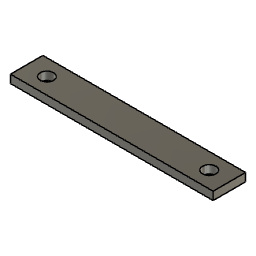
Headbar (Autodesk Fusion 360 design; units mm, degrees)
Autodesk Fusion 360 part; units mm, degrees
sketch "Sketch1" plane through (0, 0, 0) normal (0, 0, 1) x (1, 0, 0)
  line L0 (-47.1003, 10.1518) -> (-22.1003, 10.1518)
  line L1 (-22.1003, 10.1518) -> (-22.1003, 6.1518)
  line L2 (-22.1003, 6.1518) -> (-47.1003, 6.1518)
  line L3 (-47.1003, 6.1518) -> (-47.1003, 10.1518)
  circle A0 centre (-44.6003, 8.1518) radius 0.825
  circle A1 centre (-24.6003, 8.1696) radius 0.825
  line L4 (-47.1003, 8.1518) -> (-44.6003, 8.1518) construction
  line L5 (-22.1003, 8.1518) -> (-24.6003, 8.1696)
  dimension "d1" = 25
  dimension "d2" = 4
  dimension "d3" = 1.65
  dimension "d4" = 1.65
  dimension "d7" = 2.5
  dimension "d8" = 2.5
  constraint horizontal L0
  constraint vertical L1
  constraint horizontal L2
  constraint vertical L3
  constraint midpoint L3 L4.start
  constraint perpendicular L3 L4
  constraint coincident A0.centre L4.end
  constraint midpoint L1 L5.start
  constraint coincident A1.centre L5.end
  measures "d1" distance of L0.start L0.end
  measures "d2" distance of L0.start L2.end
  measures "d3" diameter of A0
  measures "d4" diameter of A1
  measures "d7" distance of L4.start A0.centre
  measures "d8" horizontal distance of L5.start A1.centre
extrude "Extrude1" add sketch "Sketch1" along normal blind 1
